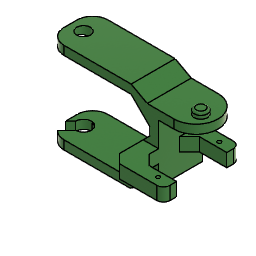
second_joint (Autodesk Fusion 360 design; units mm, degrees)
Autodesk Fusion 360 part; units mm, degrees
sketch "Sketch1" plane through (0, 0, 0) normal (0, 0, 1) x (1, 0, 0)
  line L0 (0, 0) -> (50, 0)
  line L1 (50, 0) -> (50, 20)
  line L2 (50, 20) -> (0, 20)
  line L3 (0, 20) -> (0, 0)
  line L4 (0, 10) -> (50, 10) construction
  circle A0 centre (5.9, 10) radius 3.6
  circle A1 centre (22.1, 10) radius 2.4
  line L5 (2.3, 10) -> (2.3, 19) construction
  line L6 (22.2778, 12.3934) -> (6.1667, 13.5901)
  line L7 (22.2778, 7.6066) -> (6.1667, 6.4099)
  dimension "d1" = 20
  dimension "d2" = 50
  dimension "d3" = 7.2
  dimension "d4" = 4.8
  dimension "d5" = 5.9
  dimension "d68" = 16.2
  constraint horizontal L0
  constraint vertical L1
  constraint horizontal L2
  constraint vertical L3
  constraint coincident L0.start L3.end
  constraint midpoint L3 L4.start
  constraint midpoint L1 L4.end
  constraint coincident L4 A0.centre
  constraint coincident L4 A1.centre
  constraint coincident A0 L5.start
  constraint coincident L4 L5.start
  constraint tangent A0 L5
  constraint coincident A1 L6.start
  constraint coincident A0 L6.end
  constraint tangent A1 L6
  constraint symmetric L4 L6.start L7.start
  constraint symmetric L4 L6.end L7.end
  constraint tangent A0 L6
  measures "d1" distance of L0.start L2.end
  measures "d2" distance of L1.end L2.end
  measures "d3" diameter of A0
  measures "d4" diameter of A1
  measures "d5" distance of L3 A0.centre
  measures "d68" distance of A0.centre A1.centre
extrude "Extrude1" add sketch "Sketch1" along normal blind 4 contours L0 L1 L2 L3 | A0 A1 L6 L7 | A1 makes body 1
extrude "Extrude2" cut sketch "Sketch1" along normal blind 2.5 contours A0 A1 L6 L7 | A1 bodies 1
sketch "Sketch2" plane through (0, 0, 4) normal (0, 0, 1) x (-1, 0, 0)
  circle A0 centre (-5.9, -10) radius 3.6
  line L0 (0, -20) -> (0, 0)
  line L1 (0, 0) -> (-50, 0)
  line L2 (-50, 0) -> (-50, -20)
  line L3 (-50, -20) -> (0, -20)
  line L4 (-50, -20) -> (-46, -20)
  line L5 (-46, -20) -> (-46, 0)
  line L6 (-46, 0) -> (-50, 0)
  line L7 (-50, 0) -> (-50, -20)
  dimension "d12" = 4
  constraint horizontal L4
  constraint vertical L5
  constraint horizontal L6
  constraint vertical L7
  constraint coincident L1 L5.end
  constraint coincident L2.end L3.start
  measures "d12" distance of L2.end L4.end
extrude "Extrude3" add sketch "Sketch2" along normal blind 33.2 contours L1 L2 L3 L4 L5 L6 L7 bodies 1
sketch "Sketch3" plane through (50, 0, 0) normal (1, 0, 0) x (0, 1, 0)
  line L0 (0, 0) -> (20, 0)
  line L1 (20, 0) -> (20, 37.2)
  line L2 (20, 37.2) -> (0, 37.2)
  line L3 (0, 37.2) -> (0, 0)
  line L4 (0, 37.2) -> (20, 37.2)
  line L5 (20, 37.2) -> (20, 41.2)
  line L6 (20, 41.2) -> (0, 41.2)
  line L7 (0, 41.2) -> (0, 37.2)
  dimension "d15" = 20
  dimension "d16" = 4
  constraint horizontal L4
  constraint vertical L5
  constraint horizontal L6
  constraint vertical L7
  constraint coincident L2.end L3.start
  measures "d15" distance of L2.end L1.end
  measures "d16" distance of L2.end L6.end
extrude "Extrude4" add sketch "Sketch3" against normal up to surface (50 mm away) contours L2 L4 L5 L6 L7 bodies 1
sketch "Sketch5" plane through (0, 0, 41.2) normal (0, 0, 1) x (-1, 0, 0)
  line L0 (0, -20) -> (0, 0)
  line L1 (0, 0) -> (-50, 0)
  line L2 (-50, 0) -> (-50, -20)
  line L3 (-50, -20) -> (0, -20)
  line L4 (0, -10) -> (-37, -10) construction
  circle A0 centre (-5.9, -10) radius 3.1
  dimension "d23" = 6.2
  dimension "d24" = 5.9
  constraint midpoint L0 L4.start
  constraint perpendicular L0 L4
  constraint coincident L4 A0.centre
  measures "d23" diameter of A0
  measures "d24" distance of L0 A0.centre
extrude "Extrude6" cut sketch "Sketch5" against normal blind 9 contours A0 bodies 1
sketch "Sketch6" plane through (0, 0, 0) normal (-1, 0, 0) x (0, -1, 0)
  line L0 (-20, 37.2) -> (0, 37.2)
  line L1 (0, 37.2) -> (0, 41.2)
  line L2 (0, 41.2) -> (-20, 41.2)
  line L3 (-20, 41.2) -> (-20, 37.2)
  line L4 (-10, 37.2) -> (-10, 41.2) construction
  arc A0 (-6.9, 37.2) -> (-13.1, 37.2) centre (-10, 31.8021) ccw
  dimension "d27" = 6.2
  dimension "d28" = 3.1
  constraint midpoint L0 L4.start
  constraint midpoint L2 L4.end
  constraint coincident L0 A0.end
  constraint coincident L0 A0.start
  measures "d27" distance of A0.start A0.end
  measures "d28" distance of L4.start A0.end
extrude "Extrude7" cut sketch "Sketch6" against normal blind 6 contours L0 A0 bodies 1
chamfer "Chamfer1" distance 8.5 angle 45 2 edges at (46, 10, 37.2) (46, 10, 4) on bodies 1
fillet "Fillet1" radius 7 4 edges at (0, 20, 39.2) (0, 0, 39.2) (0, 20, 2) (0, 0, 2) on bodies 1
sketch "Sketch13" plane through (50, 0, 0) normal (1, 0, 0) x (0, 1, 0)
  line L0 (0, 0) -> (20, 0)
  line L1 (20, 0) -> (20, 41.2)
  line L2 (20, 41.2) -> (0, 41.2)
  line L3 (0, 41.2) -> (0, 0)
  line L4 (20, 16) -> (14, 16)
  line L5 (14, 16) -> (14, 22)
  line L6 (14, 22) -> (20, 22)
  line L7 (20, 22) -> (20, 16)
  line L8 (-8.8, 22) -> (-14.8, 22)
  line L9 (-14.8, 22) -> (-14.8, 16)
  line L10 (-14.8, 16) -> (-8.8, 16)
  line L11 (-8.8, 16) -> (-8.8, 22)
  line L12 (20, 33.2) -> (0, 33.2)
  line L13 (0, 33.2) -> (0, 37.2)
  line L14 (0, 37.2) -> (20, 37.2)
  line L15 (20, 37.2) -> (20, 33.2)
  line L16 (20, 22) -> (-29.7229, 22) construction
  line L17 (20, 4.2) -> (0, 4.2) construction
  line L18 (-8.8, 22) -> (0, 22)
  line L19 (0, 22) -> (0, 16)
  line L20 (0, 16) -> (-8.8, 16)
  line L21 (-8.8, 16) -> (-8.8, 22)
  dimension "d71" = 6
  dimension "d72" = 6
  dimension "d74" = 6
  dimension "d75" = 22.8
  dimension "d77" = 4
  dimension "d78" = 4
  dimension "d79" = 11.2
  dimension "d80" = 6
  dimension "d81" = 29
  constraint horizontal L4
  constraint vertical L5
  constraint horizontal L6
  constraint vertical L7
  constraint coincident L1 L4.start
  constraint horizontal L8
  constraint vertical L9
  constraint horizontal L10
  constraint vertical L11
  constraint horizontal L12
  constraint vertical L13
  constraint horizontal L14
  constraint vertical L15
  constraint coincident L1 L12.start
  constraint perpendicular L7 L16
  constraint coincident L8.start L16
  constraint coincident L1 L17.start
  constraint coincident L3 L17.end
  constraint perpendicular L3 L17
  constraint horizontal L18
  constraint vertical L19
  constraint horizontal L20
  constraint vertical L21
  constraint coincident L3 L19.end
  constraint coincident L10.end L11.start
  measures "d71" distance of L5.end L6.end
  measures "d72" distance of L4.start L6.end
  measures "d74" distance of L8.start L8.end
  measures "d75" distance of L5 L11
  measures "d77" distance of L12.start L14.end
  measures "d78" distance of L2 L14
  measures "d79" distance of L6 L12
  measures "d80" distance of L8.end L9.end
  measures "d81" distance of L12 L17
extrude "Extrude14" add sketch "Sketch13" along normal blind 17 contours L1 L4 L5 L6 L7 | L8 L9 L10 L11 L21 | L1 L3 L12 L13 L14 L15 bodies 1 makes body 2 at (55.6667, -12.8, 16)
extrude "Extrude15" add sketch "Sketch13" against normal up to surface (4 mm away) contours L3 L11 L18 L19 L20 L21 | L8 L9 L10 L11 L21 bodies 1 2
sketch "Sketch14" plane through (0, 0, 16) normal (0, 0, -1) x (1, 0, 0)
  line L0 (50, 8.8) -> (67, 8.8)
  line L1 (67, 8.8) -> (67, 14.8)
  line L2 (67, 14.8) -> (46, 14.8)
  line L3 (46, 14.8) -> (46, 0)
  line L4 (46, 0) -> (50, 0)
  line L5 (50, 0) -> (50, 8.8)
  line L6 (67, -20) -> (50, -20) construction
  line L7 (67, -20) -> (67, 14.8) construction
  line L8 (67, -2.6) -> (85.3247, -2.6) construction
  circle A0 centre (61.1, 11.3) radius 0.85
  circle A1 centre (61.1, -16.5) radius 0.85
  dimension "d86" = 1.7
  dimension "d87" = 2.5
  dimension "d88" = 5.9
  constraint horizontal L6
  constraint coincident L1.end L2.start
  constraint midpoint L7 L8.start
  constraint perpendicular L7 L8
  constraint symmetric L8 A0 A1
  measures "d86" diameter of A0
  measures "d87" distance of L0 A0.centre
  measures "d88" distance of L7 A0.centre
extrude "Extrude16" cut sketch "Sketch14" against normal blind 13 contours A0 | A1 bodies 1
sketch "Sketch15" plane through (0, 0, 37.2) normal (0, 0, 1) x (-1, 0, 0)
  line L0 (-50, -20) -> (-50, 0)
  line L1 (-50, 0) -> (-67, 0)
  line L2 (-67, 0) -> (-67, -20)
  line L3 (-67, -20) -> (-50, -20)
  circle A0 centre (-61.1, -8.1) radius 3
  dimension "d91" = 6
  dimension "d92" = 11.9
  dimension "d93" = 5.9
  measures "d91" diameter of A0
  measures "d92" distance of L3 A0.centre
  measures "d93" distance of L2 A0.centre
extrude "Extrude17" add sketch "Sketch15" along normal blind 2.5 contours A0 bodies 1
chamfer "Chamfer2" distance 4.5 angle 45 1 edges at (50, -8.8, 19) on bodies 1
sketch "Sketch16" plane through (46, 0, 0) normal (-1, 0, 0) x (0, -1, 0)
  line L0 (-20, 12.5) -> (0, 12.5)
  line L1 (0, 12.5) -> (0, 16)
  line L2 (0, 16) -> (14.8, 16)
  line L3 (14.8, 16) -> (14.8, 22)
  line L4 (14.8, 22) -> (0, 22)
  line L5 (0, 22) -> (0, 28.7)
  line L6 (0, 28.7) -> (-20, 28.7)
  line L7 (-20, 28.7) -> (-20, 12.5)
  line L8 (14.8, 22) -> (-20, 22)
  line L9 (-20, 22) -> (-20, 16)
  line L10 (-20, 16) -> (14.8, 16)
  line L11 (14.8, 16) -> (14.8, 22)
  constraint horizontal L8
  constraint vertical L9
  constraint horizontal L10
  constraint vertical L11
  constraint coincident L7 L9.end
  constraint coincident L3.end L4.start
  constraint coincident L2.end L3.start
extrude "Extrude18" add sketch "Sketch16" along normal blind 3 contours L2 L3 L4 L7 L8 L9 L10 L11 bodies 1
chamfer "Chamfer3" distance 4 angle 45 1 edges at (43, -14.8, 19) on bodies 1
chamfer "Chamfer4" distance 3 angle 45 2 edges at (46, 10, 16) (46, 10, 22) on bodies 1
fillet "Fillet9" radius 3 2 edges at (67, -14.8, 19) (67, 20, 19) on bodies 1
fillet "Fillet10" radius 10 1 edges at (67, 0, 35.2) on bodies 1
fillet "Fillet11" radius 10 1 edges at (67, 20, 35.2) on bodies 1
chamfer "Chamfer5" distance 4.5 angle 45 1 edges at (50, 14, 19) on bodies 1
sketch "Sketch17" plane through (0, 0, 0) normal (0, 0, -1) x (1, 0, 0)
  line L0 (50, 0) -> (7, 0)
  arc A0 (7, 0) -> (0, -7) centre (7, -7) ccw
  line L1 (0, -7) -> (0, -13)
  arc A1 (0, -13) -> (7, -20) centre (7, -13) ccw
  line L2 (7, -20) -> (50, -20)
  line L3 (22.2778, -12.3934) -> (6.1667, -13.5901)
  arc A2 (6.1667, -6.4099) -> (6.1667, -13.5901) centre (5.9, -10) ccw
  line L4 (6.1667, -6.4099) -> (22.2778, -7.6066)
  arc A3 (22.2778, -12.3934) -> (22.2778, -7.6066) centre (22.1, -10) ccw
  line L5 (5.9, -10) -> (-4.6501, 0.5501) construction
  line L6 (5.9, -10) -> (20.8201, -10) construction
  line L7 (7.8296, -8.2526) -> (-5.7371, 5.314)
  line L8 (7.8296, -8.2526) -> (27.0157, -8.2526) construction
  line L9 (4.1526, -11.9296) -> (-9.414, 1.6371)
  line L10 (-6.9268, -0.8501) -> (-3.2499, 2.8268)
  line L11 (4.1526, -11.9296) -> (7.8296, -8.2526)
  line L12 (50, -20) -> (50, 0)
  dimension "d110" = 135
  dimension "d111" = 135
  dimension "d112" = 2.6
  dimension "d113" = -5.2
  constraint horizontal L6
  constraint coincident A2.centre L5.start
  constraint horizontal L8
  constraint coincident L9 L10.start
  constraint coincident L7 L10.end
  constraint perpendicular L7 L10
  constraint perpendicular L7 L11
  measures "d110" angle of L5 L6
  measures "d111" angle of L7 L8
  measures "d112" distance of L5 L7
extrude "Extrude19" cut sketch "Sketch17" against normal blind 9 contours A0 L1 A2 L7 L9 | A0 L1 L7 L9 L10 | A2 L7 L9 L11 bodies 1
fillet "Fillet12" radius 1 1 edges at (9.5, 10, 2.5) on bodies 1
sketch "Sketch18" plane through (0, 0, 0) normal (0, -1, 0) x (1, 0, 0)
  line L0 (57, 33.2) -> (57, 37.2)
  line L1 (57, 37.2) -> (50, 37.2)
  line L2 (50, 37.2) -> (50, 41.2)
  line L3 (50, 41.2) -> (7, 41.2)
  line L4 (7, 41.2) -> (7, 37.2)
  line L5 (7, 37.2) -> (37.5, 37.2)
  line L6 (37.5, 37.2) -> (46, 28.7)
  line L7 (46, 28.7) -> (46, 25)
  line L8 (46, 25) -> (43, 22)
  line L9 (43, 22) -> (50, 22)
  line L10 (50, 22) -> (50, 33.2)
  line L11 (50, 33.2) -> (57, 33.2)
  line L12 (7, 0) -> (50, 0)
  line L13 (50, 0) -> (50, 16)
  line L14 (50, 37.2) -> (37.5296, 37.2)
  line L15 (37.5296, 37.2) -> (37.5296, 41.2)
  line L16 (37.5296, 41.2) -> (50, 41.2)
  line L17 (50, 41.2) -> (50, 37.2)
  line L18 (50, 0) -> (37, 0)
  line L19 (37, 0) -> (37, 4)
  line L20 (37, 4) -> (50, 4)
  line L21 (50, 4) -> (50, 0)
  line L22 (37.5296, 41.2) -> (44.8249, 37.2)
  line L23 (37, 0) -> (43.5, 4)
  constraint horizontal L14
  constraint vertical L15
  constraint horizontal L16
  constraint vertical L17
  constraint coincident L3 L15.end
  constraint coincident L1.end L2.start
  constraint horizontal L18
  constraint vertical L19
  constraint horizontal L20
  constraint vertical L21
  constraint coincident L12.end L13.start
  constraint coincident L14 L22.end
  constraint midpoint L20 L23.end
extrude "Extrude20" cut sketch "Sketch18" against normal blind 25 contours L2 L3 L14 L16 L17 L22 | L12 L13 L18 L20 L21 L23 bodies 1
chamfer "Chamfer6" distance 3 angle 45 1 edges at (50, 10, 4) on bodies 1
fillet "Fillet13" radius 1 1 edges at (63.897, 9.1848, 39.7) on bodies 1
equation "d92 = 5.9 mm + 6 mm"
